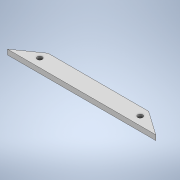
# Autodesk Inventor part: Flash
Saved by Autodesk Inventor 2020.2 (Build 242310000, 310)
## iProperties
Created: 2025-04-19
Part Number: Flash
Material: Типовые
Document SubType Name: Modeling
Designer: Кир
Density: 1 g/cm^3
Appearance: По умолчанию
Author: Кир
Autodesk Inventor part; units mm, degrees
ref_plane "YZ Plane" through (0, 0, 0) normal (1, 0, 0) x (0, 1, 0)
ref_plane "XZ Plane" through (0, 0, 0) normal (0, 1, 0) x (-1, 0, 0)
ref_plane "XY Plane" through (0, 0, 0) normal (0, 0, 1) x (1, 0, 0)
sketch "Эскиз1" plane through (0, 0, 0) normal (0, 1, 0) x (-1, 0, 0)
  line L0 (-30, -5) -> (30, -5)
  line L1 (30, -5) -> (30, 5)
  line L2 (30, 5) -> (-30, 5)
  line L3 (-30, 5) -> (-30, -5)
  line L4 (-30, -5) -> (30, 5) construction
  line L5 (30, -5) -> (-30, 5) construction
  line L6 (30, 5) -> (44.2815, 5)
  line L7 (30, -5) -> (44.2815, 5)
  line L8 (30, -5) -> (49.277, -5) construction
  line L9 (-30, 5) -> (-44.2815, 5)
  line L10 (-30, -5) -> (-44.2815, 5)
  line L11 (-30, -5) -> (0.6976, -5) construction
  circle A0 centre (30, 0) radius 1.5
  circle A1 centre (-30, 0) radius 1.5
  point P0 (0, 0)
  dimension "d0" = 60
  dimension "d1" = 10
  dimension "d3" = 35
  dimension "d4" = 145
  dimension "d7" = 3
  dimension "d8" = 3
  constraints: 24 end point, 4 midpoint, 3 horizontal, 2 centre point, 2 parallel, 1 perpendicular
  measures "d0" distance of L2.end L1.end
  measures "d1" distance of L1.end L0.end
  measures "d3" angle of L8 L7
  measures "d4" angle of L11 L10
  measures "d7" diameter of A0
  measures "d8" diameter of A1
extrude "Выдавливание1" add sketch "Эскиз1" along normal blind 3 contours L3 A1 L2 L1 A0 L0 | L10 L9 L3 A1 | L1 A0 L6 L7
